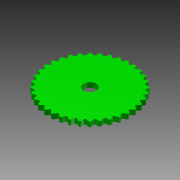
# Autodesk Inventor part: Kugghjul 5mm
Saved by Autodesk Inventor 2012 SP1 (Build 160190100, 190)
## iProperties
Created: 2014-02-18
Part Number: Kugghjul 5mm
Material: Default
Document SubType Name: Modeling
Designer: Pinkponk
Density: 1 g/cm^3
Author: Pinkponk
Autodesk Inventor part; units mm, degrees
ref_plane "YZ Plane" through (0, 0, 0) normal (1, 0, 0) x (0, 1, 0)
ref_plane "XZ Plane" through (0, 0, 0) normal (0, 1, 0) x (-1, 0, 0)
ref_plane "XY Plane" through (0, 0, 0) normal (0, 0, 1) x (1, 0, 0)
sketch "Sketch1" plane through (0, 0, 0) normal (0, 0, 1) x (1, 0, 0)
  circle A0 centre (0, 0) radius 17.5
  circle A1 centre (0, 0) radius 2.5
  dimension "d0" = 35
  dimension "d1" = 5
  constraints: 2 centre point, 2 coincident
  measures "d0" diameter of A0
  measures "d1" diameter of A1
extrude "Extrusion1" add sketch "Sketch1" along normal blind 2
sketch "Sketch2" plane through (0, 0, 2) normal (0, 0, 1) x (1, 0, 0)
  circle A0 centre (0, 0) radius 17.5 projected
  line L0 (0, 0) -> (7.3958, 15.8604) construction
  line L1 (0, 0) -> (4.5293, 16.9037) construction
  line L2 (4.5293, 16.9037) -> (5.3013, 14.5652)
  line L3 (5.3013, 14.5652) -> (7.3958, 15.8604)
  circle A1 centre (0, 0) radius 15.5 construction
  line L4 (0, 0) -> (5.3013, 14.5652) construction
  line L5 (0, 0) -> (0, 7.7829) construction
  arc A2 (7.3958, 15.8604) -> (4.5293, 16.9037) centre (0, 0) ccw
  dimension "d4" = 10
  dimension "d5" = 2
  dimension "d6" = 5
  dimension "d7" = 20
  constraints: 12 end point, 4 point on circle, 2 coincident, 2 point on line, 1 centre point, 1 vertical, 3 other
  measures "d4" angle of L1 L0
  measures "d6" angle of L0 L4
  measures "d7" angle of L5 L4
extrude "Extrusion2" cut sketch "Sketch2" against normal through all contours L3 L2 A0 picked at (5.1117, 16.0269)
pattern_circular "Circular Pattern1" count 36 over 360 about axis through (0, 0, 0) along (0, 0, 1) of "Extrusion2"
fillet "Fillet1" radius 0.5 2 edges at (5.3013, 14.5652, 1) (4.5293, 16.9037, 1)
pattern_circular "Circular Pattern2" count 36 over 360 about axis through (0, 0, 0) along (0, 0, 1) of "Fillet1"
body "Solid1"
